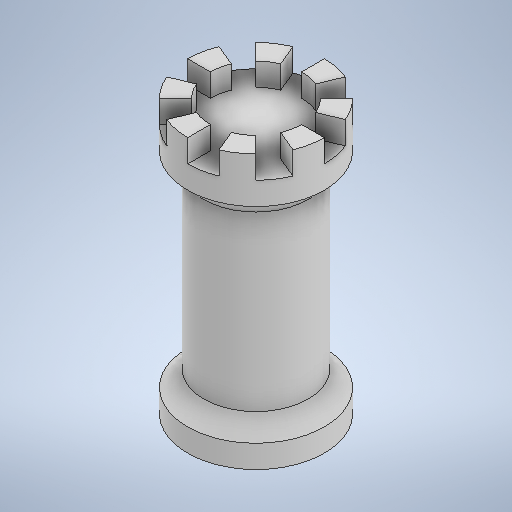
# Autodesk Inventor part: TowerUntagged
Saved by Autodesk Inventor 2025.2 (Build 292293000, 293)
## iProperties
Created: 2025-02-26
Part Number: TowerUntagged
Material: Generic
Document SubType Name: Modeling
Designer: Marcu
Density: 1 g/cm^3
Appearance: Default
Author: Marcu
Autodesk Inventor part; units mm, degrees
ref_plane "YZ Plane" through (0, 0, 0) normal (1, 0, 0) x (0, 1, 0)
ref_plane "XZ Plane" through (0, 0, 0) normal (0, 1, 0) x (-1, 0, 0)
ref_plane "XY Plane" through (0, 0, 0) normal (0, 0, 1) x (1, 0, 0)
sketch "Sketch1" plane through (0, 0, 0) normal (0, 1, 0) x (-1, 0, 0)
  circle A0 centre (0, 0) radius 15
  dimension "d0" = 30
  constraints: 1 centre point, 1 coincident
  measures "d0" diameter of A0
extrude "Extrusion1" add sketch "Sketch1" along normal blind 60
sketch "Sketch2" plane through (0, 60, 0) normal (0, 1, 0) x (1, 0, 0)
  arc A0 (-3.8268, -9.2388) -> (0, -10) centre (0, 0) ccw
  line L0 (0, -10) -> (0, -15)
  circle A1 centre (0, 0) radius 15 projected
  line L1 (-3.8268, -9.2388) -> (-5.7403, -13.8582)
  arc A2 (-5.7403, -13.8582) -> (0, -15) centre (0, 0) ccw
  arc A3 (3.8268, -9.2388) -> (7.0711, -7.0711) centre (0, 0) ccw
  line L2 (7.0711, -7.0711) -> (10.6066, -10.6066)
  line L3 (3.8268, -9.2388) -> (5.7403, -13.8582)
  arc A4 (5.7403, -13.8582) -> (10.6066, -10.6066) centre (0, 0) ccw
  arc A5 (9.2388, -3.8268) -> (10, 0) centre (0, 0) ccw
  line L4 (10, 0) -> (15, 0)
  line L5 (9.2388, -3.8268) -> (13.8582, -5.7403)
  arc A6 (13.8582, -5.7403) -> (15, 0) centre (0, 0) ccw
  arc A7 (9.2388, 3.8268) -> (7.0711, 7.0711) centre (0, 0) ccw
  line L6 (7.0711, 7.0711) -> (10.6066, 10.6066)
  line L7 (9.2388, 3.8268) -> (13.8582, 5.7403)
  arc A8 (13.8582, 5.7403) -> (10.6066, 10.6066) centre (0, 0) ccw
  arc A9 (3.8268, 9.2388) -> (0, 10) centre (0, 0) ccw
  line L8 (0, 10) -> (0, 15)
  line L9 (3.8268, 9.2388) -> (5.7403, 13.8582)
  arc A10 (5.7403, 13.8582) -> (0, 15) centre (0, 0) ccw
  arc A11 (-3.8268, 9.2388) -> (-7.0711, 7.0711) centre (0, 0) ccw
  line L10 (-7.0711, 7.0711) -> (-10.6066, 10.6066)
  line L11 (-3.8268, 9.2388) -> (-5.7403, 13.8582)
  arc A12 (-5.7403, 13.8582) -> (-10.6066, 10.6066) centre (0, 0) ccw
  arc A13 (-9.2388, 3.8268) -> (-10, 0) centre (0, 0) ccw
  line L12 (-10, 0) -> (-15, 0)
  line L13 (-9.2388, 3.8268) -> (-13.8582, 5.7403)
  arc A14 (-13.8582, 5.7403) -> (-15, 0) centre (0, 0) ccw
  arc A15 (-9.2388, -3.8268) -> (-7.0711, -7.0711) centre (0, 0) ccw
  line L14 (-7.0711, -7.0711) -> (-10.6066, -10.6066)
  line L15 (-9.2388, -3.8268) -> (-13.8582, -5.7403)
  arc A16 (-13.8582, -5.7403) -> (-10.6066, -10.6066) centre (0, 0) ccw
  point P0 (15, 0)
  dimension "d3" = 20
  dimension "d7" = 360
  constraints: 34 point on circle, 32 end point, 16 centre point, 2 coincident, 1 vertical, 81 other
  measures "d3" diameter of A0
extrude "Extrusion2" cut sketch "Sketch2" against normal blind 5 contours L1 A1 L14 A15 L15 L12 A13 L13 L10 A11 L11 L8 A9 L9 L6 A7 L7 L4 A5 L5 L2 A3 L3 L0 A0
sketch "Sketch3" plane through (0, 0, 0) normal (1, 0, 0) x (0, 1, 0)
  line L0 (0, 15) -> (60, 15) projected
  line L1 (55, -13.8582) -> (55, -15) projected
  line L2 (0, -15) -> (60, -15) projected
  line L3 (50, -15) -> (46.4645, -11.4645)
  line L4 (0, -15) -> (0, 15) projected
  line L5 (0, -15) -> (5, -15)
  line L6 (5, -15) -> (8.5355, -11.4645)
  line L7 (8.5355, -11.4645) -> (46.4645, -11.4645)
  line L8 (46.4645, -11.4645) -> (8.5355, -11.4645)
  line L9 (50, -15) -> (50, -20)
  line L10 (50, -20) -> (5, -20)
  line L11 (5, -20) -> (5, -15)
  line L12 (0, 0) -> (62.9673, 0)
  dimension "d13" = 5
  dimension "d16" = 5
  dimension "d17" = 5
  constraints: 18 end point, 3 perpendicular, 3 point on line, 2 parallel, 1 horizontal
  measures "d13" distance of L3.start L3.end
  measures "d16" distance of L5.end L6.end
  measures "d17" distance of L3.start L9.end
revolve "Revolution1" cut sketch "Sketch3" angle 360 about axis through (0, 0, 0) along (0, 1, 0)
sketch "Sketch4" plane through (0, 0, 0) normal (0, -1, 0) x (1, 0, 0)
  circle A0 centre (0, 0) radius 11.4645 projected
  circle A1 centre (0, 0) radius 2.5
  dimension "d19" = 5
  constraints: 1 centre point, 1 coincident
  measures "d19" diameter of A1
extrude "Extrusion3" cut sketch "Sketch4" against normal blind 4 contours A1
body "Solid1"
